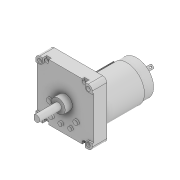
# Autodesk Inventor part: Orange MG555 12V 100RPM Square Gearbox DC motor
Saved by Autodesk Inventor 2021 (Build 250183000, 183)
## iProperties
Created: 2020-01-07
Part Number: Orange MG555 12V 100RPM Square Gearbox DC motor
Material: Generic
Document SubType Name: Modeling
Designer: Johnson Ebenezer R
Density: 1 g/cm^3
Appearance: Default
Author: Johnson Ebenezer R
Autodesk Inventor part; units mm, degrees
ref_plane "YZ Plane" through (0, 0, 0) normal (1, 0, 0) x (0, 1, 0)
ref_plane "XZ Plane" through (0, 0, 0) normal (0, 1, 0) x (-1, 0, 0)
sketch "Sketch1" plane through (0, 0, 0) normal (0, 0, 1) x (1, 0, 0)
  line L0 (-35, -35) -> (35, -35)
  line L1 (35, -35) -> (35, 35)
  line L2 (35, 35) -> (-35, 35)
  line L3 (-35, 35) -> (-35, -35)
  line L4 (-35, -35) -> (35, 35) construction
  line L5 (35, -35) -> (-35, 35) construction
  point P0 (0, 0)
  dimension "d0" = 70
  constraints: 12 end point, 2 midpoint, 2 parallel, 2 perpendicular, 1 horizontal
  measures "d0" distance of L1.end L2.end
extrude "Extrusion1" add sketch "Sketch1" against normal blind 18
fillet "Fillet1" radius 5 4 edges at (-35, 35, -9) (35, 35, -9) (35, -35, -9) (-35, -35, -9)
sketch "Sketch2" plane through (0, 0, 0) normal (0, 0, 1) x (1, 0, 0)
  line L0 (-35, -30) -> (-35, 30) construction
  line L1 (-35, 0) -> (35, 0) construction
  line L2 (35, 30) -> (35, -30) construction
  line L3 (-30, 35) -> (30, 35) construction
  line L4 (0, 35) -> (0, -35) construction
  line L5 (30, -35) -> (-30, -35) construction
  circle A0 centre (-30, 30) radius 2.5
  line L6 (-35, 26.3) -> (-30, 26.3)
  line L7 (-26.3, 30) -> (-26.3, 35)
  arc A1 (-30, 26.3) -> (-26.3, 30) centre (-30, 30) ccw
  circle A2 centre (30, 30) radius 2.5
  line L8 (35, 26.3) -> (30, 26.3)
  line L9 (26.3, 30) -> (26.3, 35)
  arc A3 (26.3, 30) -> (30, 26.3) centre (30, 30) ccw
  circle A4 centre (-30, -30) radius 2.5
  line L10 (-35, -26.3) -> (-30, -26.3)
  line L11 (-26.3, -30) -> (-26.3, -35)
  arc A5 (-26.3, -30) -> (-30, -26.3) centre (-30, -30) ccw
  circle A6 centre (30, -30) radius 2.5
  line L12 (26.3, -30) -> (26.3, -35)
  arc A7 (30, -26.3) -> (26.3, -30) centre (30, -30) ccw
  line L13 (35, -26.3) -> (30, -26.3)
  line L14 (-26.3, 35) -> (26.3, 35)
  line L15 (35, 26.3) -> (35, -26.3)
  line L16 (26.3, -35) -> (-26.3, -35)
  line L17 (-35, -26.3) -> (-35, 26.3)
  point P0 (0, 0)
  dimension "d5" = 5
  dimension "d6" = 5
  dimension "d7" = 5
  dimension "d9" = 1.2
  constraints: 28 end point, 18 symmetric about line, 8 centre point, 8 point on circle, 4 midpoint, 3 collinear, 3 perpendicular, 2 point on line, 2 tangent, 1 concentric, 6 other
  measures "d5" distance from line of A0.centre L3
  measures "d6" distance from line of A0.centre L0
  measures "d7" diameter of A0
  measures "d9" radial gap between concentric circles of A1 A0
extrude "Extrusion2" cut sketch "Sketch2" against normal blind 2
sketch "Sketch3" plane through (0, 0, 0) normal (0, 0, 1) x (1, 0, 0)
  arc A0 (-26.3, -30) -> (-30, -26.3) centre (-30, -30) ccw projected
  circle A1 centre (-30, 30) radius 2.5 projected
  circle A2 centre (30, 30) radius 2.5 projected
  circle A3 centre (30, -30) radius 2.5 projected
  point P0 (0, 0)
  constraints: 4 coincident
hole "Hole1" at (-30, -30, 0) at (-30, 30, 0) at (30, 30, 0) at (30, -30, 0) direction (0, 0, -1) diameter 3.9 depth 20 counterbore diameter 5 counterbore depth 7.2
sketch "Sketch4" plane through (0, 0, -2) normal (0, 0, 1) x (1, 0, 0)
  line L0 (-30, 35) -> (30, 35) construction
  line L1 (0, 35) -> (0, -35) construction
  line L2 (26.3, -35) -> (-26.3, -35) construction
  line L3 (-35, -26.3) -> (-35, 26.3) construction
  line L4 (-35, 0) -> (35, 0) construction
  line L5 (35, 30) -> (35, -30) construction
  line L6 (-20.6, 35) -> (-20.6, 32.85)
  line L7 (-20.6, 32.85) -> (-26.3, 32.85) construction
  line L8 (-26.3, 30) -> (-26.3, 35) projected
  line L9 (-26.3, 35) -> (-26.3, 32.85)
  line L10 (-26.3, 35) -> (-20.6, 35)
  arc A0 (-26.3, 32.85) -> (-20.6, 32.85) centre (-23.45, 32.85) ccw
  line L11 (-23.45, 30) -> (-23.45, 35) construction
  line L12 (30, 35) -> (-30, 35) construction
  line L13 (20.6, 35) -> (20.6, 32.85)
  line L14 (20.6, 32.85) -> (26.3, 32.85) construction
  line L15 (26.3, 30) -> (26.3, 35)
  line L16 (26.3, 35) -> (26.3, 32.85)
  line L17 (26.3, 35) -> (20.6, 35)
  arc A1 (20.6, 32.85) -> (26.3, 32.85) centre (23.45, 32.85) ccw
  line L18 (23.45, 30) -> (23.45, 35) construction
  line L19 (-30, -35) -> (30, -35) construction
  line L20 (-20.6, -35) -> (-20.6, -32.85)
  line L21 (-20.6, -32.85) -> (-26.3, -32.85) construction
  line L22 (-26.3, -30) -> (-26.3, -35)
  line L23 (-26.3, -35) -> (-26.3, -32.85)
  line L24 (-26.3, -35) -> (-20.6, -35)
  arc A2 (-20.6, -32.85) -> (-26.3, -32.85) centre (-23.45, -32.85) ccw
  line L25 (-23.45, -30) -> (-23.45, -35) construction
  line L26 (30, -35) -> (-30, -35) construction
  line L27 (20.6, -35) -> (20.6, -32.85)
  line L28 (23.45, -30) -> (23.45, -35) construction
  line L29 (20.6, -32.85) -> (26.3, -32.85) construction
  line L30 (26.3, -30) -> (26.3, -35)
  line L31 (26.3, -35) -> (26.3, -32.85)
  line L32 (26.3, -35) -> (20.6, -35)
  arc A3 (26.3, -32.85) -> (20.6, -32.85) centre (23.45, -32.85) ccw
  point P0 (0, 0)
  dimension "d19" = 5.7
  dimension "d21" = 5
  constraints: 56 end point, 33 symmetric about line, 12 point on line, 9 point on circle, 5 midpoint, 4 centre point, 2 perpendicular, 2 tangent, 1 collinear, 1 vertical, 3 other
  measures "d19" distance between parallel lines of L8 L6
  measures "d21" distance of L11.start L11.end
extrude "Extrusion3" cut sketch "Sketch4" against normal blind 3
sketch "Sketch5" plane through (0, 0, -2) normal (0, 0, 1) x (1, 0, 0)
  circle A0 centre (0, 0) radius 8.5
  dimension "d24" = 17
  constraints: 1 centre point, 1 coincident
  measures "d24" diameter of A0
extrude "Extrusion4" add sketch "Sketch5" along normal blind 9
sketch "Sketch6" plane through (0, 0, 7) normal (0, 0, 1) x (1, 0, 0)
  circle A0 centre (0, 0) radius 4
  line L0 (-3, 2.6458) -> (-3, -2.6458)
  line L1 (-3, 0) -> (4, 0) construction
  dimension "d27" = 8
  dimension "d28" = 7
  constraints: 4 end point, 3 point on circle, 1 centre point, 1 coincident, 1 horizontal, 1 midpoint, 1 vertical
  measures "d27" diameter of A0
  measures "d28" distance of L1.start L1.end
extrude "Extrusion5" add sketch "Sketch6" along normal blind 27 contours A0 L0 picked at (0.3596, 0.8073)
sketch "Sketch7" plane through (0, 0, -2) normal (0, 0, 1) x (1, 0, 0)
  circle A0 centre (-19, -7.5) radius 3.1
  circle A1 centre (-17, -23.5) radius 3
  circle A2 centre (-5, -25.5) radius 2.6
  circle A3 centre (7, -24.5) radius 2.5
  circle A4 centre (14, -14.5) radius 3
  line L0 (-35, -26.3) -> (-35, 26.3) projected
  line L1 (20.6, -35) -> (-20.6, -35) projected
  line L2 (35, 26.3) -> (35, -26.3) projected
  point P0 (0, 0)
  dimension "d31" = 6.2
  dimension "d32" = 16
  dimension "d33" = 27.5
  dimension "d34" = 6
  dimension "d35" = 18
  dimension "d36" = 11.5
  dimension "d37" = 5.2
  dimension "d38" = 9.5
  dimension "d39" = 30
  dimension "d40" = 5
  dimension "d41" = 10.5
  dimension "d42" = 28
  dimension "d43" = 6
  dimension "d44" = 21
  dimension "d45" = 20.5
  constraints: 5 centre point
  measures "d31" diameter of A0
  measures "d32" distance from line of A0.centre L0
  measures "d33" distance from line of A0.centre L1
  measures "d34" diameter of A1
  measures "d35" distance from line of A1.centre L0
  measures "d36" distance from line of A1.centre L1
  measures "d37" diameter of A2
  measures "d38" distance from line of A2.centre L1
  measures "d39" distance from line of A2.centre L0
  measures "d40" diameter of A3
  measures "d41" distance from line of A3.centre L1
  measures "d42" distance from line of L2 A3.centre
  measures "d43" diameter of A4
  measures "d44" distance from line of A4.centre L2
  measures "d45" distance from line of A4.centre L1
extrude "Extrusion6" add sketch "Sketch7" along normal blind 2
sketch "Sketch8" plane through (0, 0, -18) normal (0, 0, -1) x (-1, 0, 0)
  circle A0 centre (0, -17.75) radius 17.25
  line L0 (-30, -35) -> (30, -35) projected
  circle A1 centre (13.0767, -29) radius 2.5
  line L1 (-12.1976, -29.9476) -> (12.1976, -5.5524) construction
  circle A2 centre (-11.25, -4.6733) radius 2.5
  circle A3 centre (0, 2) radius 9.25
  line L2 (0, -35) -> (0, 11.25)
  circle A4 centre (-24.25, 7) radius 4.5
  circle A5 centre (-24.25, -17) radius 4.5
  circle A6 centre (24.25, 7) radius 4.5
  circle A7 centre (24.25, -17) radius 4.5
  line L3 (-24.25, 7) -> (24.25, 7) construction
  line L4 (30, 35) -> (-30, 35) projected
  point P0 (0, 0)
  point P1 (0, 7)
  point P2 (-8.0772, -2.5079)
  point P3 (-9.2417, -3.1845)
  point P4 (-13.022, -6.4368)
  point P5 (11.3132, -30.772)
  point P6 (14.5655, -26.9917)
  point P7 (8.0772, -2.5079)
  dimension "d52" = 18.5
  dimension "d48" = 34.5
  dimension "d49" = 5
  dimension "d50" = 6
  dimension "d51" = 45
  dimension "d53" = 37
  dimension "d54" = 48.5
  dimension "d55" = 24
  dimension "d56" = 9
  dimension "d57" = 28
  constraints: 7 centre point, 6 end point, 5 vertical alignment, 4 point on circle, 3 equal radius, 3 midpoint, 2 horizontal alignment, 1 coincident, 1 horizontal, 1 perpendicular, 1 symmetric about line, 4 other
  measures "d48" diameter of A0
  measures "d49" diameter of A1
  measures "d50" distance from line of A1.centre L0
  measures "d51" angle of L1 L0
  measures "d53" distance from line of point (0, 2) L0
  measures "d54" distance of L3.start L3.end
  measures "d55" distance of A7.centre L3.end
  measures "d56" diameter of A4
  measures "d57" distance between parallel lines of L4 L3
extrude "Extrusion7" add sketch "Sketch8" along normal blind 5.5
sketch "Sketch9" plane through (0, 0, -23.5) normal (0, 0, -1) x (-1, 0, 0)
  arc A0 (14.5655, -26.9917) -> (8.0772, -2.5079) centre (0, -17.75) ccw projected
  circle A1 centre (0, -17.75) radius 21
  point P0 (0, 0)
  dimension "d60" = 42
  constraints: 1 centre point, 1 coincident
  measures "d60" diameter of A1
extrude "Extrusion8" add sketch "Sketch9" along normal blind 66.5
sketch "Sketch10" plane through (0, 0, 0) normal (1, 0, 0) x (0, 1, 0)
  line L0 (-14.2307, -23.5) -> (1.1234, -23.5) projected
  line L1 (-1.75, -23.5) -> (-1.75, -28.5) construction
  line L2 (3.25, -23.5) -> (3.25, -90) projected
  arc A0 (3.25, -28.5) -> (-1.75, -23.5) centre (-1.75, -28.5) ccw
  line L3 (-1.75, -28.5) -> (3.25, -28.5) construction
  line L4 (-38.75, -90) -> (3.25, -90) projected
  line L5 (-17.75, -90) -> (-17.75, -23.5)
  line L6 (-1.75, -23.5) -> (3.25, -23.5)
  line L7 (1.1234, -23.5) -> (11.25, -23.5) projected
  line L8 (3.25, -28.5) -> (3.25, -23.5)
  point P0 (0, 0)
  point P1 (1.1234, -23.5)
  dimension "d63" = 5
  dimension "d64" = 5
  dimension "d65" = 5
  constraints: 10 end point, 2 point on circle, 2 point on line, 2 vertical, 1 centre point, 1 collinear, 1 horizontal, 1 midpoint, 1 perpendicular
  measures "d63" radius of A0
  measures "d64" distance of L1.start L1.end
  measures "d65" distance of L1.end L3.end
revolve "Revolution1" cut sketch "Sketch10" angle 360 about axis through (0, -17.75, -90) along (0, 0, 1)
ref_plane "Work Plane1" through (0, -17.75, -28.5) normal (0, 0, -1) x (-1, 0, 0)
sketch "Sketch11" plane through (0, -17.75, -28.5) normal (0, 0, -1) x (-1, 0, 0)
  circle A0 centre (0, 0) radius 21 projected
  circle A1 centre (0, 0) radius 13.6692
  circle A2 centre (0, 0) radius 22.2
  line L0 (0, 0) -> (10.0786, 19.7803)
  line L1 (0, -17.25) -> (30, -17.25) projected
  line L2 (0, 0) -> (15.6978, 15.6978)
  line L3 (15.6978, 15.6978) -> (10.0786, 19.7803)
  point P0 (0, 17.75)
  point P1 (9.5338, 18.7111)
  point P2 (14.8492, 14.8492)
  dimension "d67" = 44.4
  dimension "d68" = 63
  dimension "d69" = 45
  constraints: 6 end point, 2 centre point, 2 coincident, 2 point on circle
  measures "d67" diameter of A2
  measures "d68" angle of L0 L1
  measures "d69" angle of L2 L1
extrude "Extrusion9" add sketch "Sketch11" along normal blind 49 contours A0 L2 A2 L1 | L1 A2 L0 A0
sketch "Sketch12" plane through (0, 0, 0) normal (1, 0, 0) x (0, 1, 0)
  line L0 (-38.75, -90) -> (3.25, -90) projected
  line L1 (-17.75, -90) -> (-17.75, -98.5) construction
  line L2 (-10.25, -90) -> (-10.25, -92.6716)
  arc A0 (-12.25, -95.5) -> (-10.25, -92.6716) centre (-13.25, -92.6716) ccw
  line L3 (-12.25, -95.5) -> (-14.25, -96.5)
  line L4 (-14.25, -96.5) -> (-15.25, -96.5)
  line L5 (-15.25, -96.5) -> (-15.25, -98)
  arc A1 (-17.75, -98.5) -> (-15.25, -98) centre (-17.75, -92) ccw
  line L6 (-17.75, -98.5) -> (-15.25, -98.5) construction
  line L7 (-17.75, -98.5) -> (-17.75, -90)
  line L8 (-10.25, -90) -> (-17.75, -90)
  point P0 (0, 0)
  dimension "d72" = 3
  dimension "d73" = 2
  dimension "d74" = 2.5
  dimension "d75" = 7.5
  dimension "d76" = 1
  dimension "d77" = 1
  dimension "d78" = 6.5
  dimension "d79" = 2
  dimension "d80" = 1.5
  constraints: 16 end point, 4 point on circle, 2 centre point, 2 horizontal, 2 perpendicular, 2 point on line, 2 tangent, 2 vertical, 1 collinear, 1 midpoint, 1 vertical alignment
  measures "d72" radius of A0
  measures "d73" horizontal distance of L3.end L3.start
  measures "d74" distance between parallel lines of L5 L1
  measures "d75" distance between parallel lines of L2 L1
  measures "d76" distance of L3.end L4.end
  measures "d77" vertical distance of L3.end L3.start
  measures "d78" distance between parallel lines of L0 L4
  measures "d79" distance from line of L6.start L4
  measures "d80" distance of L4.end L5.end
revolve "Revolution2" add sketch "Sketch12" angle 360 about axis through (0, -17.75, -98.5) along (0, 0, 1)
sketch "Sketch13" plane through (0, -17.75, -90) normal (0, 0, -1) x (-1, 0, 0)
  arc A0 (9.5338, 18.7111) -> (14.8492, 14.8492) centre (0, 0) ccw projected
  line L0 (-13.4985, 16.0869) -> (0, 0) construction
  line L1 (0, 0) -> (-16.9601, -14.2312) construction
  line L2 (-30, -17.25) -> (0, -17.25) projected
  line L3 (-13.4087, 12.2461) -> (-9.7317, 15.3315)
  line L4 (-9.7317, 15.3315) -> (-9.3781, 14.9102)
  line L5 (-9.3781, 14.9102) -> (-13.0552, 11.8248)
  line L6 (-13.0552, 11.8248) -> (-13.4087, 12.2461)
  line L7 (9.7317, -15.3315) -> (13.4087, -12.2461)
  line L8 (13.4087, -12.2461) -> (13.0552, -11.8248)
  line L9 (13.0552, -11.8248) -> (9.3781, -14.9102)
  line L10 (9.3781, -14.9102) -> (9.7317, -15.3315)
  point P0 (0, 17.75)
  point P1 (-11.5702, 13.7888)
  dimension "d83" = 50
  dimension "d84" = 3
  dimension "d85" = 0.55
  dimension "d86" = 4.8
  constraints: 20 end point, 4 perpendicular, 4 symmetric about line, 1 midpoint, 1 parallel, 1 point on circle, 1 point on line
  measures "d83" angle of L0 L2
  measures "d84" distance from line of L0.start L3
  measures "d85" distance between parallel lines of L3 L5
  measures "d86" distance between parallel lines of L4 L6
extrude "Extrusion10" add sketch "Sketch13" along normal blind 8.5
sketch "Sketch14" plane through (13.4087, -5.5039, -90) normal (0.6427876, 0.7660444, 0) x (0.7660444, -0.6427876, 0)
  line L0 (-9.9, 0) -> (5.1, 0) projected
  line L1 (-4.3, 0) -> (-4.3, 1.5)
  line L2 (-4.3, 1.5) -> (-4.8, 1.5)
  line L3 (-4.8, 0) -> (-4.8, 8.5) projected
  line L4 (-4.8, 7.5) -> (-4.3, 8.5)
  line L5 (-4.8, 8.5) -> (0, 8.5) projected
  line L6 (-0.5, 8.5) -> (0, 7.5)
  line L7 (-4.8, 0) -> (0, 0) projected
  line L8 (-0.5, 0) -> (-0.5, 1.5)
  line L9 (-0.5, 1.5) -> (0, 1.5)
  line L10 (0, 0) -> (0, 8.5) projected
  line L11 (-2.4, 5) -> (-2.4, 6) construction
  line L12 (-4.8, 0) -> (-4.8, 8.5) projected
  line L13 (-1.45, 5) -> (-1.45, 6)
  line L14 (-3.35, 6) -> (-3.35, 5)
  arc A0 (-3.35, 5) -> (-1.45, 5) centre (-2.4, 5) ccw
  arc A1 (-1.45, 6) -> (-3.35, 6) centre (-2.4, 6) ccw
  line L15 (-2.4, 4.05) -> (-2.4, 6.95) construction
  point P0 (-13.8095, -90)
  point P1 (-2.4, 5.5)
  point P2 (-2.4, 8.5)
  point P3 (-0.5, 0)
  dimension "d89" = 1.5
  dimension "d90" = 0.5
  dimension "d91" = 0.5
  dimension "d92" = 1
  dimension "d93" = 3
  dimension "d95" = 1.9
  dimension "d96" = 2.9
  constraints: 22 end point, 8 point on line, 6 point on circle, 4 tangent, 3 vertical alignment, 2 centre point, 2 horizontal alignment, 2 midpoint, 2 parallel, 2 perpendicular, 2 vertical
  measures "d89" distance between parallel lines of L0 L2
  measures "d90" distance between parallel lines of L3 L1
  measures "d91" distance between parallel lines of L8 L10
  measures "d92" distance from line of L4.start L5
  measures "d93" distance from line of L5 point (-2.4, 5.5)
  measures "d95" distance between parallel lines of L14 L13
  measures "d96" distance of L15.start L15.end
extrude "Extrusion11" cut sketch "Sketch14" against normal blind 8.5 contours L3 L2 L1 L0 | L8 L9 L10 L0 | L3 L5 L4 | L5 L10 L6 | A0 L14 A1 L13
sketch "Sketch15" plane through (-9.3781, -32.6602, -90) normal (0.6427876, 0.7660444, 0) x (0.7660444, -0.6427876, 0)
  line L0 (-10.0107, 0) -> (4.9893, 0)
  line L1 (-4.3, 0) -> (-4.3, 1.5)
  line L2 (-4.3, 1.5) -> (-4.8, 1.5)
  line L3 (-4.8, 0) -> (-4.8, 8.5)
  line L4 (-4.8, 7.5) -> (-4.3, 8.5)
  line L5 (-4.8, 8.5) -> (0, 8.5)
  line L6 (-0.5, 8.5) -> (0, 7.5)
  line L7 (-4.8, 0) -> (0, 0)
  line L8 (-0.5, 0) -> (-0.5, 1.5)
  line L9 (-0.5, 1.5) -> (0, 1.5)
  line L10 (0, 0) -> (0, 8.5)
  line L11 (-2.4, 5) -> (-2.4, 6) construction
  line L12 (-4.8, 0) -> (-4.8, 8.5)
  line L13 (-1.45, 5) -> (-1.45, 6)
  line L14 (-3.35, 6) -> (-3.35, 5)
  arc A0 (-3.35, 5) -> (-1.45, 5) centre (-2.4, 5) ccw
  arc A1 (-1.45, 6) -> (-3.35, 6) centre (-2.4, 6) ccw
  line L15 (-2.4, 4.05) -> (-2.4, 6.95) construction
  line L16 (0, 0) -> (-4.8, 0) projected
  line L17 (-4.8, 8.5) -> (0, 8.5) projected
  point P0 (-13.8095, -90)
  point P1 (-13.8095, -90)
  point P2 (-2.4, 5.5)
  point P3 (-2.4, 8.5)
  point P4 (-0.5, 0)
  point P5 (-2.4, 0)
  point P6 (-0.5, 0)
  dimension "d99" = 1.5
  dimension "d100" = 0.5
  dimension "d101" = 0.5
  dimension "d102" = 1
  dimension "d103" = 3
  dimension "d104" = 1.9
  dimension "d105" = 2.9
  constraints: 34 end point, 9 point on line, 6 point on circle, 4 tangent, 3 midpoint, 3 vertical alignment, 2 centre point, 2 horizontal alignment, 2 parallel, 2 perpendicular, 2 vertical, 1 collinear
  measures "d99" distance between parallel lines of L0 L2
  measures "d100" distance between parallel lines of L3 L1
  measures "d101" distance between parallel lines of L8 L10
  measures "d102" distance from line of L4.start L5
  measures "d103" distance from line of L5 point (-2.4, 5.5)
  measures "d104" distance between parallel lines of L14 L13
  measures "d105" distance of L15.start L15.end
extrude "Extrusion12" cut sketch "Sketch15" against normal blind 8.5 contours L3 L2 L1 L0 | L8 L9 L10 L0 | L3 L5 L4 | L5 L10 L6 | A0 L14 A1 L13
body "Solid1"
